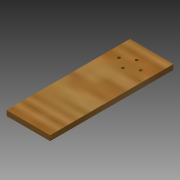
# Autodesk Inventor part: segment3a
Saved by Autodesk Inventor 2013 (Build 170138000, 138)
## iProperties
Created: 2014-10-12
Part Number: segment3a
Material: Plywood, Finish
Document SubType Name: Modeling
Designer: Masta
Density: 1 g/cm^3
Author: Masta
Autodesk Inventor part; units mm, degrees
ref_plane "YZ Plane" through (0, 0, 0) normal (1, 0, 0) x (0, 1, 0)
ref_plane "XZ Plane" through (0, 0, 0) normal (0, 1, 0) x (-1, 0, 0)
ref_plane "XY Plane" through (0, 0, 0) normal (0, 0, 1) x (1, 0, 0)
sketch "Sketch1" plane through (0, 0, 0) normal (0, 0, 1) x (1, 0, 0)
  line L0 (0, 0) -> (-7.5, 0) construction
  line L1 (0, 0) -> (0, 4.75) construction
  line L2 (0, 0) -> (0, 15)
  line L3 (0, 15) -> (-15, 15)
  line L4 (-15, 15) -> (-15, -70)
  line L5 (-15, -70) -> (0, -70)
  line L6 (0, -70) -> (0, 0)
  dimension "d10" = 7.5
  dimension "d14" = 4.75
  dimension "d17" = 15
  dimension "d18" = 15
  dimension "d19" = 70
  constraints: 14 end point, 4 coincident, 2 collinear, 2 parallel, 2 perpendicular, 1 horizontal
  measures "d10" distance of L0.start L0.end
  measures "d14" distance of point (0, 4.75) point (0, 0)
  measures "d17" distance of L0.start L2.end
  measures "d18" distance of L2.end L3.end
  measures "d19" distance of L5.end L0.start
extrude "Extrusion1" add sketch "Sketch1" along normal blind 3.5
hole "Hole1" at (0, 4.75, 0) at (-7.5, 0, 0) direction (0, 0, 1) diameter 2 end through all
mirror "Mirror2" about plane through (0, 0, 0) normal (0, 1, 0) of "Hole1"
mirror "Mirror1" about plane through (0, 0, 0) normal (1, 0, 0)
body "Solid1"
